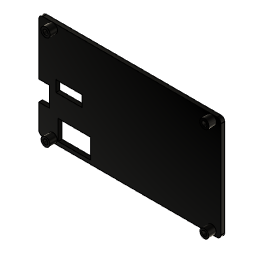
Fysetc_5i_LCD_for_Voron_V1.8 (Autodesk Fusion 360 archive; units mm, degrees)
design "Fysetc_5i_LCD_Back_MacNite"
Autodesk Fusion 360 part; units mm, degrees
sketch "Sketch1" plane through (0, 0, 0) normal (0, 1, 0) x (1, 0, 0)
  line L0 (0, 0) -> (127.4, 0) construction
  line L1 (127.4, 0) -> (127.4, -76.2) construction
  line L2 (127.4, -76.2) -> (0, -76.2) construction
  line L3 (0, -76.2) -> (0, 0) construction
  circle A0 centre (0, -76.2) radius 2
  circle A1 centre (127.4, -76.2) radius 2
  circle A2 centre (127.4, 0) radius 2
  circle A3 centre (0, 0) radius 2
  line L4 (2.2, -76.7) -> (125.2, -76.7)
  line L5 (125.2, -76.7) -> (125.2, 3)
  line L6 (125.2, 3) -> (2.2, 3)
  line L7 (2.2, 3) -> (2.2, -76.7)
  line L8 (-11.8, -80.45) -> (135.2, -80.45)
  line L9 (135.2, -80.45) -> (135.2, 4)
  line L10 (135.2, 4) -> (-11.8, 4)
  line L11 (-11.8, 4) -> (-11.8, -80.45)
  line L12 (137.2, 6) -> (-13.8, 6)
  line L13 (-13.8, 6) -> (-13.8, -82.45)
  line L14 (-13.8, -82.45) -> (137.2, -82.45)
  line L15 (137.2, -82.45) -> (137.2, 6)
  line L16 (8.4, -74.8) -> (120, -74.8)
  line L17 (120, -74.8) -> (120, -5.9)
  line L18 (120, -5.9) -> (8.4, -5.9)
  line L19 (8.4, -5.9) -> (8.4, -74.8)
  dimension "d1" = 76.2
  dimension "d2" = 127.4
  dimension "d3" = 4
  dimension "d4" = 4
  dimension "d5" = 4
  dimension "d6" = 4
  dimension "d8" = 123
  dimension "d9" = 0.5
  dimension "d10" = 3
  dimension "d11" = 2.2
  dimension "d12" = 3.75
  dimension "d13" = 1
  dimension "d14" = 14
  dimension "d15" = 10
  dimension "d16" = 2
  dimension "d22" = 1.9
  dimension "d23" = 8.9
  dimension "d24" = 6.2
  dimension "d25" = 5.2
  constraint horizontal L0
  constraint vertical L1
  constraint horizontal L2
  constraint vertical L3
  constraint coincident L0.start L3.end
  constraint coincident L2.end L3.start
  constraint coincident L1.end L2.start
  constraint coincident L0.end L1.start
  constraint horizontal L4
  constraint vertical L5
  constraint horizontal L6
  constraint vertical L7
  constraint horizontal L8
  constraint vertical L9
  constraint horizontal L10
  constraint vertical L11
  constraint horizontal L16
  constraint vertical L17
  constraint horizontal L18
  constraint vertical L19
  measures "d1" distance of L0.start L2.end
  measures "d2" distance of L0.start L0.end
  measures "d3" diameter of A0
  measures "d4" diameter of A1
  measures "d5" diameter of A2
  measures "d6" diameter of A3
  measures "d8" distance of L4.start L4.end
  measures "d9" distance of L2.end L4
  measures "d10" distance of L0.start L6
  measures "d11" distance of L0.start L7
  measures "d12" distance of L4 L8
  measures "d13" distance of L6 L10
  measures "d14" distance of L7 L11
  measures "d15" distance of L5 L9
  measures "d22" distance of L4 L16
  measures "d23" distance of L6 L18
  measures "d24" distance of L7 L19
  measures "d25" distance of L5 L17
extrude "Extrude1" add sketch "Sketch1" along normal blind 3 contours L4 L5 L6 L7 | L8 L9 L10 L11 | L16 L17 L18 L19
sketch "Sketch2" plane through (0, 0, 0) normal (0, -1, 0) x (1, 0, 0)
  circle A0 centre (0, 0) radius 2
  circle A1 centre (127.4, 76.2) radius 2
  circle A2 centre (127.4, 0) radius 2
  circle A3 centre (0, 76.2) radius 2
  line L0 (-11.8, 80.45) -> (-11.8, -4)
  line L1 (-11.8, -4) -> (135.2, -4)
  line L2 (135.2, -4) -> (135.2, 80.45)
  line L3 (135.2, 80.45) -> (-11.8, 80.45)
  line L4 (-11.3, -3.5) -> (134.7, -3.5)
  line L5 (134.7, -3.5) -> (134.7, 79.95)
  line L6 (134.7, 79.95) -> (-11.3, 79.95)
  line L7 (-11.3, 79.95) -> (-11.3, -3.5)
  circle A4 centre (0, 76.2) radius 3.75
  circle A5 centre (0, 0) radius 3.5
  circle A6 centre (127.4, 0) radius 3.5
  circle A7 centre (127.4, 76.2) radius 3.75
  dimension "d29" = -0.5
  constraint concentric A3 A4
  constraint concentric A0 A5
  constraint concentric A2 A6
  constraint concentric A1 A7
  constraint tangent L6 A4
  constraint tangent L6 A7
  constraint tangent L4 A6
  constraint tangent L4 A5
extrude "Extrude4" add sketch "Sketch2" along normal blind 6 contours A5 | A6 | A7 | A4
extrude "Extrude12" cut sketch "Sketch2" against normal blind 6 contours L0 L1 L2 L3
fillet "Fillet2" radius 3 4 edges at (-11.3, 1.5, -3.5) (134.7, 1.5, -3.5) (134.7, 1.5, 79.95) (-11.3, 1.5, 79.95)
sketch "Sketch3" plane through (0, 0, 0) normal (0, -1, 0) x (1, 0, 0)
  circle A0 centre (0, 0) radius 3.5
  circle A1 centre (0, 76.2) radius 3.75
  circle A2 centre (127.4, 0) radius 3.5
  circle A3 centre (127.4, 76.2) radius 3.75
  line L0 (30.2, -0.6) -> (4.2, -0.6)
  line L1 (4.2, -0.6) -> (4.2, 15.4)
  line L2 (4.2, 15.4) -> (30.2, 15.4)
  line L3 (30.2, 15.4) -> (30.2, -0.6)
  line L4 (-11.8, 19) -> (-2.8, 19)
  line L5 (-2.8, 19) -> (-2.8, 35)
  line L6 (-2.8, 35) -> (-11.8, 35)
  line L7 (-11.8, 35) -> (-11.8, 19)
  line L8 (23.4, 32.5) -> (2.4, 32.5)
  line L9 (2.4, 32.5) -> (2.4, 41.5)
  line L10 (2.4, 41.5) -> (23.4, 41.5)
  line L11 (23.4, 41.5) -> (23.4, 32.5)
  line L12 (86.45, 38.225) -> (36.95, 38.225) construction
  circle A4 centre (36.95, 38.225) radius 1.5
  circle A5 centre (86.45, 38.225) radius 1.5
  line L13 (-8.3, -3.5) -> (0, -3.5)
  line L14 (134.7, -0.5) -> (134.7, 76.95)
  line L15 (131.7, 79.95) -> (127.4, 79.95)
  line L16 (127.4, 79.95) -> (0, 79.95)
  line L17 (-11.3, 76.95) -> (-11.3, -0.5)
  arc A6 (-8.3, 79.95) -> (-11.3, 76.95) centre (-8.3, 76.95) ccw
  arc A7 (-11.3, -0.5) -> (-8.3, -3.5) centre (-8.3, -0.5) ccw
  line L18 (0, -3.5) -> (127.4, -3.5)
  line L19 (127.4, -3.5) -> (131.7, -3.5)
  arc A8 (131.7, -3.5) -> (134.7, -0.5) centre (131.7, -0.5) ccw
  arc A9 (134.7, 76.95) -> (131.7, 79.95) centre (131.7, 76.95) ccw
  line L20 (0, 79.95) -> (-8.3, 79.95)
  dimension "d33" = 26
  dimension "d34" = 16
  dimension "d36" = 4.2
  dimension "d38" = 16
  dimension "d39" = 9
  dimension "d42" = 21
  dimension "d43" = 9
  dimension "d44" = 49.5
  dimension "d45" = 3
  dimension "d46" = 3
  constraint horizontal L0
  constraint vertical L1
  constraint horizontal L2
  constraint vertical L3
  constraint horizontal L4
  constraint vertical L5
  constraint horizontal L6
  constraint vertical L7
  constraint horizontal L8
  constraint vertical L9
  constraint horizontal L10
  constraint vertical L11
  constraint horizontal L12
  constraint coincident L12.end A4.centre
  constraint coincident L12.start A5.centre
  measures "d33" distance of L0.start L0.end
  measures "d34" distance of L0.start L2.end
  measures "d36" distance of A0.centre L1
  measures "d38" distance of L4.end L5.end
  measures "d39" distance of L4.start L4.end
  measures "d42" distance of L8.start L8.end
  measures "d43" distance of L8.start L10.end
  measures "d44" distance of L12.start L12.end
  measures "d45" diameter of A4
  measures "d46" diameter of A5
extrude "Extrude5" cut sketch "Sketch3" against normal through all contours L4 L5 L6 L17 | L4 L6 L7 L17 | L0 L1 L2 L3 | L8 L9 L10 L11
sketch "Sketch4" plane through (0, 3, 0) normal (0, 1, 0) x (-1, 0, 0)
  line L0 (2.8, 35) -> (11.3, 35)
  line L1 (11.3, 19) -> (2.8, 19)
  line L2 (2.8, 19) -> (2.8, 35)
  line L3 (-4.2, 15.4) -> (-4.2, -0.6)
  line L4 (-4.2, -0.6) -> (-30.2, -0.6)
  line L5 (-30.2, -0.6) -> (-30.2, 15.4)
  line L6 (-30.2, 15.4) -> (-4.2, 15.4)
  line L7 (-2.4, 41.5) -> (-2.4, 32.5)
  line L8 (-2.4, 32.5) -> (-23.4, 32.5)
  line L9 (-23.4, 32.5) -> (-23.4, 41.5)
  line L10 (-23.4, 41.5) -> (-2.4, 41.5)
  circle A0 centre (0, 0) radius 2
  circle A1 centre (-127.4, 76.2) radius 2
  circle A2 centre (-127.4, 0) radius 2
  circle A3 centre (0, 76.2) radius 2
  line L11 (-75.45, 48.225) -> (-47.95, 48.225)
  line L12 (-47.95, 48.225) -> (-47.95, 28.225)
  line L13 (-47.95, 28.225) -> (-75.45, 28.225)
  line L14 (-75.45, 28.225) -> (-75.45, 48.225)
  line L15 (11.3, 35) -> (11.3, 76.95)
  line L16 (8.3, 79.95) -> (-131.7, 79.95)
  line L17 (-134.7, 76.95) -> (-134.7, -0.5)
  line L18 (-131.7, -3.5) -> (8.3, -3.5)
  arc A4 (11.3, 76.95) -> (8.3, 79.95) centre (8.3, 76.95) ccw
  arc A5 (-131.7, 79.95) -> (-134.7, 76.95) centre (-131.7, 76.95) ccw
  arc A6 (-134.7, -0.5) -> (-131.7, -3.5) centre (-131.7, -0.5) ccw
  arc A7 (8.3, -3.5) -> (11.3, -0.5) centre (8.3, -0.5) ccw
  line L19 (11.3, -0.5) -> (11.3, 19)
  constraint horizontal L11
  constraint vertical L12
  constraint horizontal L13
  constraint vertical L14
extrude "Extrude6" add sketch "Sketch4" along normal blind 2 contours L11 L12 L13 L14
sketch "Sketch5" plane through (0, 5, 0) normal (0, 1, 0) x (-1, 0, 0)
  line L0 (-75.45, 28.225) -> (-47.95, 28.225)
  line L1 (-47.95, 28.225) -> (-47.95, 48.225)
  line L2 (-47.95, 48.225) -> (-75.45, 48.225)
  line L3 (-75.45, 48.225) -> (-75.45, 28.225)
  line L4 (-47.95, 48.225) -> (-45.95, 48.225)
  line L5 (-45.95, 48.225) -> (-45.95, 28.225)
  line L6 (-45.95, 28.225) -> (-47.95, 28.225)
  line L7 (-47.95, 28.225) -> (-47.95, 48.225)
  line L8 (-75.45, 48.225) -> (-77.45, 48.225)
  line L9 (-77.45, 48.225) -> (-77.45, 28.225)
  line L10 (-77.45, 28.225) -> (-75.45, 28.225)
  line L11 (-75.45, 28.225) -> (-75.45, 48.225)
  dimension "d59" = 2
  dimension "d60" = 2
  constraint horizontal L4
  constraint vertical L5
  constraint horizontal L6
  constraint vertical L7
  constraint coincident L1.end L2.start
  constraint coincident L0.end L6
  constraint horizontal L8
  constraint vertical L9
  constraint horizontal L10
  constraint vertical L11
  constraint coincident L2.end L3.start
  constraint coincident L0.start L10
  measures "d59" distance of L2.end L8.end
  measures "d60" distance of L1.end L4.end
extrude "Extrude7" add sketch "Sketch5" along normal blind 3
chamfer "Chamfer2" distance 2 angle 45 2 edges at (45.95, 5, 38.225) (77.45, 5, 38.225)
sketch "Sketch8" plane through (0, 3, 0) normal (0, 1, 0) x (-1, 0, 0)
  line L0 (-75.45, 28.225) -> (-75.45, 48.225)
  line L1 (-75.45, 48.225) -> (-47.95, 48.225)
  line L2 (-47.95, 48.225) -> (-47.95, 28.225)
  line L3 (-47.95, 28.225) -> (-75.45, 28.225)
  line L4 (2.8, 35) -> (11.3, 35)
  line L5 (11.3, 19) -> (2.8, 19)
  line L6 (2.8, 19) -> (2.8, 35)
  line L7 (-23.4, 32.5) -> (-23.4, 41.5)
  line L8 (-23.4, 41.5) -> (-2.4, 41.5)
  line L9 (-2.4, 41.5) -> (-2.4, 32.5)
  line L10 (-2.4, 32.5) -> (-23.4, 32.5)
  line L11 (-30.2, -0.6) -> (-30.2, 15.4)
  line L12 (-30.2, 15.4) -> (-4.2, 15.4)
  line L13 (-4.2, 15.4) -> (-4.2, -0.6)
  line L14 (-4.2, -0.6) -> (-30.2, -0.6)
  circle A0 centre (0, 0) radius 2
  circle A1 centre (-127.4, 76.2) radius 2
  circle A2 centre (-127.4, 0) radius 2
  circle A3 centre (0, 76.2) radius 2
  line L15 (-50.45, 30.725) -> (-72.95, 30.725)
  line L16 (-72.95, 30.725) -> (-72.95, 45.725)
  line L17 (-72.95, 45.725) -> (-50.45, 45.725)
  line L18 (-50.45, 45.725) -> (-50.45, 30.725)
  line L19 (11.3, 35) -> (11.3, 76.95)
  line L20 (8.3, 79.95) -> (-131.7, 79.95)
  line L21 (-134.7, 76.95) -> (-134.7, -0.5)
  line L22 (-131.7, -3.5) -> (8.3, -3.5)
  arc A4 (11.3, 76.95) -> (8.3, 79.95) centre (8.3, 76.95) ccw
  arc A5 (-131.7, 79.95) -> (-134.7, 76.95) centre (-131.7, 76.95) ccw
  arc A6 (-134.7, -0.5) -> (-131.7, -3.5) centre (-131.7, -0.5) ccw
  arc A7 (8.3, -3.5) -> (11.3, -0.5) centre (8.3, -0.5) ccw
  line L23 (11.3, -0.5) -> (11.3, 19)
  dimension "d69" = 2.5
extrude "Extrude10" cut sketch "Sketch8" along normal blind 5 contours L0 L1 L2 L3 | L4 L5 L6 L19 L20 L21 L22 A4 A5 A6 A7 L23 | L15 L16 L17 L18
extrude "Extrude11" cut sketch "Sketch8" against normal blind 6 contours L15 L16 L17 L18
sketch "Sketch9" plane through (0, 0, 0) normal (0, -1, 0) x (1, 0, 0)
  line L0 (72.95, 45.725) -> (72.95, 30.725)
  line L1 (72.95, 30.725) -> (50.45, 30.725)
  line L2 (50.45, 30.725) -> (50.45, 45.725)
  line L3 (50.45, 45.725) -> (72.95, 45.725)
  line L4 (-11.3, 35) -> (-2.8, 35)
  line L5 (-2.8, 35) -> (-2.8, 19)
  line L6 (-2.8, 19) -> (-11.3, 19)
  line L7 (-11.3, 19) -> (-11.3, -0.5)
  arc A0 (-11.3, -0.5) -> (-8.3, -3.5) centre (-8.3, -0.5) ccw
  line L8 (-8.3, -3.5) -> (0, -3.5)
  circle A1 centre (0, 0) radius 3.5
  line L9 (0, -3.5) -> (127.4, -3.5)
  circle A2 centre (127.4, 0) radius 3.5
  line L10 (127.4, -3.5) -> (131.7, -3.5)
  arc A3 (131.7, -3.5) -> (134.7, -0.5) centre (131.7, -0.5) ccw
  line L11 (134.7, -0.5) -> (134.7, 76.95)
  arc A4 (134.7, 76.95) -> (131.7, 79.95) centre (131.7, 76.95) ccw
  line L12 (131.7, 79.95) -> (127.4, 79.95)
  circle A5 centre (127.4, 76.2) radius 3.75
  line L13 (127.4, 79.95) -> (0, 79.95)
  circle A6 centre (0, 76.2) radius 3.75
  line L14 (0, 79.95) -> (-8.3, 79.95)
  arc A7 (-8.3, 79.95) -> (-11.3, 76.95) centre (-8.3, 76.95) ccw
  line L15 (-11.3, 76.95) -> (-11.3, 35)
  line L16 (30.2, 15.4) -> (30.2, -0.6)
  line L17 (30.2, -0.6) -> (4.2, -0.6)
  line L18 (4.2, -0.6) -> (4.2, 15.4)
  line L19 (4.2, 15.4) -> (30.2, 15.4)
  line L20 (23.4, 41.5) -> (23.4, 32.5)
  line L21 (23.4, 32.5) -> (2.4, 32.5)
  line L22 (2.4, 32.5) -> (2.4, 41.5)
  line L23 (2.4, 41.5) -> (23.4, 41.5)
  line L24 (50.45, 30.725) -> (72.95, 30.725)
  line L25 (72.95, 30.725) -> (72.95, 25.725)
  line L26 (72.95, 25.725) -> (50.45, 25.725)
  line L27 (50.45, 25.725) -> (50.45, 30.725)
  line L28 (50.45, 45.725) -> (72.95, 45.725)
  line L29 (72.95, 45.725) -> (72.95, 40.725)
  line L30 (72.95, 40.725) -> (50.45, 40.725)
  line L31 (50.45, 40.725) -> (50.45, 45.725)
  dimension "d77" = 5
  dimension "d78" = 5
  constraint horizontal L24
  constraint vertical L25
  constraint horizontal L26
  constraint vertical L27
  constraint coincident L1.end L2.start
  constraint horizontal L28
  constraint vertical L29
  constraint horizontal L30
  constraint vertical L31
  constraint coincident L2.end L3.start
  constraint coincident L0.start L29
  constraint coincident L0.end L25
  measures "d77" distance of L0.start L29.end
  measures "d78" distance of L1.end L26.end
extrude "Extrude13" cut sketch "Sketch9" against normal blind 6 contours L1 L24 L25 L26 L27
extrude "Extrude14" add sketch "Sketch9" against normal up to surface (3 mm away) contours L0 L2 L3 L28 L29 L30 L31
sketch "Sketch10" plane through (0, 0, 0) normal (0, -1, 0) x (1, 0, 0)
  line L0 (23.4, 41.5) -> (23.4, 32.5)
  line L1 (23.4, 32.5) -> (2.4, 32.5)
  line L2 (2.4, 32.5) -> (2.4, 41.5)
  line L3 (2.4, 41.5) -> (23.4, 41.5)
  line L4 (30.2, 15.4) -> (30.2, -0.6)
  line L5 (30.2, -0.6) -> (4.2, -0.6)
  line L6 (4.2, -0.6) -> (4.2, 15.4)
  line L7 (4.2, 15.4) -> (30.2, 15.4)
  line L8 (-11.3, 35) -> (-2.8, 35)
  line L9 (-2.8, 35) -> (-2.8, 19)
  line L10 (-2.8, 19) -> (-11.3, 19)
  line L11 (-11.3, 19) -> (-11.3, -0.5)
  arc A0 (-11.3, -0.5) -> (-8.3, -3.5) centre (-8.3, -0.5) ccw
  line L12 (-8.3, -3.5) -> (0, -3.5)
  circle A1 centre (0, 0) radius 3.5
  line L13 (0, -3.5) -> (127.4, -3.5)
  circle A2 centre (127.4, 0) radius 3.5
  line L14 (127.4, -3.5) -> (131.7, -3.5)
  arc A3 (131.7, -3.5) -> (134.7, -0.5) centre (131.7, -0.5) ccw
  line L15 (134.7, -0.5) -> (134.7, 76.95)
  arc A4 (134.7, 76.95) -> (131.7, 79.95) centre (131.7, 76.95) ccw
  line L16 (131.7, 79.95) -> (127.4, 79.95)
  circle A5 centre (127.4, 76.2) radius 3.75
  line L17 (127.4, 79.95) -> (0, 79.95)
  circle A6 centre (0, 76.2) radius 3.75
  line L18 (0, 79.95) -> (-8.3, 79.95)
  arc A7 (-8.3, 79.95) -> (-11.3, 76.95) centre (-8.3, 76.95) ccw
  line L19 (-11.3, 76.95) -> (-11.3, 35)
  line L20 (72.95, 40.725) -> (72.95, 25.725)
  line L21 (72.95, 25.725) -> (50.45, 25.725)
  line L22 (50.45, 25.725) -> (50.45, 40.725)
  line L23 (50.45, 40.725) -> (72.95, 40.725)
extrude "Extrude15" add sketch "Sketch10" against normal up to surface (3 mm away) contours L20 L21 L22 L23
equation "d60 = d59"
equation "d78 = d77"
